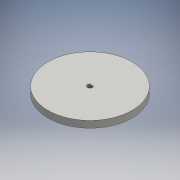
# Autodesk Inventor part: wheel
Saved by Autodesk Inventor 2016 (Build 200138000, 138)
## iProperties
Created: 2016-04-07
Part Number: wheel
Material: Generic
Document SubType Name: Modeling
Designer: hesaon
Density: 1 g/cm^3
Appearance: Default
Author: hesaon
Autodesk Inventor part; units mm, degrees
ref_plane "YZ Plane" through (0, 0, 0) normal (1, 0, 0) x (0, 1, 0)
ref_plane "XZ Plane" through (0, 0, 0) normal (0, 1, 0) x (-1, 0, 0)
ref_plane "XY Plane" through (0, 0, 0) normal (0, 0, 1) x (1, 0, 0)
sketch "Sketch1" plane through (0, 0, 0) normal (0, 0, 1) x (1, 0, 0)
  circle A0 centre (0, 0) radius 25
  arc A1 (-1.118, 1) -> (1.118, 1) centre (0, 0) ccw
  line L0 (0, 1) -> (1.118, 1)
  line L1 (1.118, 1) -> (0, 1)
  line L2 (0, 1) -> (-1.118, 1)
  dimension "d0" = 50
  dimension "d3" = 1
  dimension "d4" = 1.5
  dimension "d5" = 2.2361
  dimension "d6" = 1.118
  constraints: 6 end point, 2 centre point, 2 coincident, 2 point on circle, 1 collinear, 1 horizontal
  measures "d0" diameter of A0
  measures "d3" distance of L0.start point (0, 0)
  measures "d4" radius of A1
  measures "d5" distance of L0.end L2.end
  measures "d6" horizontal distance of point (0, 0) L2.end
extrude "Extrusion1" add sketch "Sketch1" along normal blind 4
body "Solid1"
